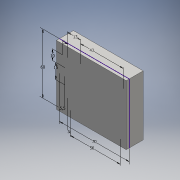
# Autodesk Inventor part: Bund
Saved by Autodesk Inventor 2016 (Build 200138000, 138)
## iProperties
Created: 2016-12-11
Part Number: Bund
Material: Generic
Document SubType Name: Modeling
Designer: Simon
Density: 1 g/cm^3
Appearance: Default
Author: Simon
Autodesk Inventor part; units mm, degrees
ref_plane "YZ Plane" through (0, 0, 0) normal (1, 0, 0) x (0, 1, 0)
ref_plane "XZ Plane" through (0, 0, 0) normal (0, 1, 0) x (-1, 0, 0)
ref_plane "XY Plane" through (0, 0, 0) normal (0, 0, 1) x (1, 0, 0)
sketch "Sketch1" plane through (0, 0, 0) normal (0, 1, 0) x (-1, 0, 0)
  line L0 (-35, 30) -> (35, 30)
  line L1 (35, 30) -> (35, -30)
  line L2 (35, -30) -> (-35, -30)
  line L3 (-35, -30) -> (-35, 30)
  line L4 (-35, 30) -> (35, -30) construction
  line L5 (35, 30) -> (-35, -30) construction
  line L6 (35, 0) -> (29.5, 0)
  line L7 (29.5, 7.5) -> (29.5, -7.5)
  line L8 (32, 7.5) -> (27, 7.5)
  line L9 (27, 7.5) -> (27, 17.5)
  line L10 (27, 17.5) -> (32, 17.5)
  line L11 (32, 17.5) -> (32, 7.5)
  line L12 (32, -7.5) -> (27, -7.5)
  line L13 (27, -7.5) -> (27, -17.5)
  line L14 (27, -17.5) -> (32, -17.5)
  line L15 (32, -17.5) -> (32, -7.5)
  line L16 (24, -26.5931) -> (-26, -26.5931)
  line L17 (-26, -26.5931) -> (-26, -4.9442)
  line L18 (-26, -4.9442) -> (24, -4.9442)
  line L19 (24, -4.9442) -> (24, -26.5931)
  line L20 (14, 18.3642) -> (-29, 18.3642)
  line L21 (-29, 18.3642) -> (-29, 5.4077)
  line L22 (-29, 5.4077) -> (14, 5.4077)
  line L23 (14, 5.4077) -> (14, 18.3642)
  point P0 (0, 0)
  dimension "d0" = 70
  dimension "d1" = 60
  dimension "d2" = 5.5
  dimension "d3" = 15
  dimension "d5" = 10
  dimension "d6" = 5
  dimension "d11" = 50
  dimension "d12" = 3
  dimension "d13" = 43
  dimension "d14" = 13
  constraints: 48 end point, 10 parallel, 6 horizontal, 6 midpoint, 5 perpendicular, 2 equal length, 1 vertical
  measures "d0" distance of L1.end L2.end
  measures "d1" distance of L0.end L1.end
  measures "d2" distance of L6.end L6.start
  measures "d3" distance of L7.start L7.end
  measures "d5" distance of L10.end L8.start
  measures "d6" distance of L9.end L10.end
  measures "d11" distance of L16.start L16.end
  measures "d12" distance between parallel lines of L13 L19
  measures "d13" distance of L20.start L20.end
  measures "d14" distance between parallel lines of L23 L9
extrude "Extrusion1" add sketch "Sketch1" along normal blind 14
extrude "Extrusion2" add sketch "Sketch1" against normal blind 3 contours L0 L1 L2 L3 | L8 L9 L10 L11 | L15 L14 L13 L12 | L16 L17 L18 L19 | L23 L22 L21 L20
body "Solid1"
